Autodesk Inventor part; units mm, degrees
(part 8 of 16)
  spline S46 degree 3 poles (26.1268, 48.1258) (26.0078, 48.1893) (25.8897, 48.2544) (25.7727, 48.3215) (25.7094, 48.3577) (25.6465, 48.3945) (25.5839, 48.4318) (25.5246, 48.4672) (25.4656, 48.5031) (25.407, 48.5395) (25.3517, 48.5739) (25.2966, 48.6087) (25.2419, 48.6441) (25.1905, 48.6773) (25.1393, 48.711) (25.0884, 48.7451) (25.0408, 48.7771) (24.9935, 48.8095) (24.9464, 48.8423) (24.9026, 48.8729) (24.859, 48.9039) (24.8156, 48.9352) (24.7755, 48.9643) (24.7356, 48.9937) (24.6959, 49.0235) (24.6594, 49.051) (24.6231, 49.0788) (24.5871, 49.1069) (24.5541, 49.1326) (24.5213, 49.1586) (24.4888, 49.1849) (24.4593, 49.2088) (24.43, 49.2329) (24.401, 49.2573) (24.3749, 49.2791) (24.349, 49.3012) (24.3233, 49.3236) (24.2894, 49.3531) (24.2559, 49.3832) (24.2226, 49.4135) (24.2152, 49.4202) (24.2077, 49.427) (24.2002, 49.4338) (24.1929, 49.4403) (24.1855, 49.4468) (24.178, 49.4532) (24.1707, 49.4595) (24.1634, 49.4657) (24.156, 49.4719) (24.1487, 49.4779) (24.1414, 49.4839) (24.1341, 49.4898) (24.1268, 49.4956) (24.1195, 49.5013) (24.1122, 49.5069) (24.105, 49.5125) (24.0977, 49.518) (24.0903, 49.5234) (24.0831, 49.5287) (24.0757, 49.5339) (24.0684, 49.5391) (24.061, 49.5442) (24.0537, 49.5492) (24.0462, 49.5541) (24.0388, 49.559) (24.0313, 49.5638) (24.0238, 49.5685) (24.0162, 49.5732) (24.0086, 49.5778) (24.0009, 49.5823) (23.9931, 49.5868) (23.9853, 49.5912) (23.9774, 49.5955) (23.9693, 49.5998) (23.9612, 49.604) (23.953, 49.608) (23.9445, 49.6122) (23.936, 49.6162) (23.9274, 49.6199) (23.9184, 49.6239) (23.9093, 49.6276) (23.9002, 49.6312) (23.8906, 49.6349) (23.8808, 49.6384) (23.871, 49.6416) (23.8605, 49.645) (23.8498, 49.6481) (23.8391, 49.6509) (23.8275, 49.654) (23.8157, 49.6566) (23.8039, 49.6588) (23.7908, 49.6612) (23.7777, 49.6632) (23.7645, 49.6645) (23.7498, 49.666) (23.735, 49.6669) (23.7201, 49.667) (23.7035, 49.6671) (23.6868, 49.6663) (23.6703, 49.6646) (23.6516, 49.6626) (23.6331, 49.6595) (23.6149, 49.6552) (23.5947, 49.6504) (23.5748, 49.6441) (23.5555, 49.6364) (23.5345, 49.628) (23.5141, 49.6181) (23.4949, 49.6064) (23.4765, 49.5952) (23.4591, 49.5824) (23.4419, 49.5693) (23.3571, 49.5047) (23.2781, 49.4332) (23.1957, 49.3657) (23.1134, 49.2982) (23.0277, 49.2348) (22.9477, 49.1643) (22.9315, 49.15) (22.9156, 49.1355) (22.901, 49.1197) (22.8857, 49.1031) (22.872, 49.0851) (22.8597, 49.0661) (22.8483, 49.0487) (22.8383, 49.0304) (22.8296, 49.0115) (22.8217, 48.9945) (22.815, 48.977) (22.8095, 48.9591) (22.8045, 48.9432) (22.8005, 48.927) (22.7973, 48.9107) (22.7945, 48.8961) (22.7924, 48.8815) (22.791, 48.8667) (22.7898, 48.8535) (22.7891, 48.8402) (22.7889, 48.827) (22.7887, 48.8149) (22.789, 48.8029) (22.7897, 48.7909) (22.7903, 48.7798) (22.7913, 48.7688) (22.7926, 48.7578) (22.7938, 48.7475) (22.7953, 48.7373) (22.7971, 48.7271) (22.7987, 48.7175) (22.8006, 48.7078) (22.8027, 48.6983) (22.8048, 48.6891) (22.807, 48.6799) (22.8094, 48.6708) (22.8117, 48.662) (22.8142, 48.6532) (22.8169, 48.6444) (22.8195, 48.6358) (22.8223, 48.6273) (22.8252, 48.6188) (22.8281, 48.6103) (22.8311, 48.602) (22.8342, 48.5936) (22.8373, 48.5853) (22.8406, 48.577) (22.8439, 48.5688) (22.8473, 48.5605) (22.8508, 48.5523) (22.8543, 48.5441) (22.8579, 48.5359) (22.8616, 48.5277) (22.8654, 48.5195) (22.8693, 48.5113) (22.8732, 48.503) (22.8772, 48.4948) (22.8813, 48.4865) (22.8855, 48.4783) (22.8898, 48.47) (22.8941, 48.4616) (22.8985, 48.4533) (22.903, 48.445) (22.9076, 48.4365) (22.9123, 48.4281) (22.917, 48.4197) (22.9218, 48.4112) (22.9267, 48.4026) (22.9317, 48.3941) (22.9368, 48.3855) (22.942, 48.3769) (22.9472, 48.3682) (22.9704, 48.3297) (22.9933, 48.2909) (23.0156, 48.2518) (23.0324, 48.2223) (23.049, 48.1925) (23.0653, 48.1626) (23.0835, 48.1294) (23.1014, 48.0959) (23.119, 48.0623) (23.1384, 48.0253) (23.1575, 47.988) (23.1762, 47.9506) (23.1967, 47.9098) (23.2168, 47.8687) (23.2366, 47.8275) (23.258, 47.7828) (23.279, 47.7379) (23.2997, 47.6928) (23.3219, 47.6442) (23.3437, 47.5953) (23.3651, 47.5463) (23.388, 47.4937) (23.4105, 47.4409) (23.4325, 47.388) (23.456, 47.3314) (23.4789, 47.2746) (23.5014, 47.2176) (23.5253, 47.1571) (23.5487, 47.0962) (23.5715, 47.0352) (23.5957, 46.9706) (23.6193, 46.9057) (23.6423, 46.8407) (23.6667, 46.7719) (23.6904, 46.703) (23.7135, 46.6338) (23.7562, 46.5059) (23.7969, 46.3773) (23.8357, 46.2482) knots 0 0 0 0 0.057795 0.057795 0.057795 0.089038 0.089038 0.089038 0.118617 0.118617 0.118617 0.14653 0.14653 0.14653 0.172778 0.172778 0.172778 0.19736 0.19736 0.19736 0.220277 0.220277 0.220277 0.241529 0.241529 0.241529 0.261115 0.261115 0.261115 0.279036 0.279036 0.279036 0.295292 0.295292 0.295292 0.309882 0.309882 0.309882 0.329164 0.329164 0.329164 0.333477 0.333477 0.333477 0.337694 0.337694 0.337694 0.34182 0.34182 0.34182 0.345864 0.345864 0.345864 0.349834 0.349834 0.349834 0.353742 0.353742 0.353742 0.3576 0.3576 0.3576 0.361424 0.361424 0.361424 0.365232 0.365232 0.365232 0.369048 0.369048 0.369048 0.372899 0.372899 0.372899 0.376819 0.376819 0.376819 0.380853 0.380853 0.380853 0.385052 0.385052 0.385052 0.389482 0.389482 0.389482 0.394225 0.394225 0.394225 0.399381 0.399381 0.399381 0.405067 0.405067 0.405067 0.411413 0.411413 0.411413 0.418548 0.418548 0.418548 0.426565 0.426565 0.426565 0.435472 0.435472 0.435472 0.445133 0.445133 0.445133 0.45436 0.45436 0.45436 0.5 0.5 0.5 0.54564 0.54564 0.54564 0.554867 0.554867 0.554867 0.564528 0.564528 0.564528 0.573435 0.573435 0.573435 0.581452 0.581452 0.581452 0.588587 0.588587 0.588587 0.594933 0.594933 0.594933 0.600619 0.600619 0.600619 0.605775 0.605775 0.605775 0.610518 0.610518 0.610518 0.614948 0.614948 0.614948 0.619147 0.619147 0.619147 0.623181 0.623181 0.623181 0.627101 0.627101 0.627101 0.630952 0.630952 0.630952 0.634768 0.634768 0.634768 0.638576 0.638576 0.638576 0.6424 0.6424 0.6424 0.646258 0.646258 0.646258 0.650166 0.650166 0.650166 0.654136 0.654136 0.654136 0.65818 0.65818 0.65818 0.662306 0.662306 0.662306 0.666523 0.666523 0.666523 0.670836 0.670836 0.670836 0.690118 0.690118 0.690118 0.704708 0.704708 0.704708 0.720964 0.720964 0.720964 0.738885 0.738885 0.738885 0.758471 0.758471 0.758471 0.779723 0.779723 0.779723 0.80264 0.80264 0.80264 0.827222 0.827222 0.827222 0.85347 0.85347 0.85347 0.881383 0.881383 0.881383 0.910962 0.910962 0.910962 0.942205 0.942205 0.942205 1 1 1 1
  arc A248 (26.1268, 48.1258) -> (26.9842, 48.907) centre (0.0435, 77.6158) ccw
  spline S47 degree 3 poles (29.0665, 51.0139) (28.9415, 51.0645) (28.8172, 51.1169) (28.6938, 51.1714) (28.6271, 51.2008) (28.5607, 51.2308) (28.4945, 51.2614) (28.4319, 51.2904) (28.3695, 51.3199) (28.3073, 51.35) (28.2487, 51.3784) (28.1903, 51.4073) (28.1322, 51.4367) (28.0776, 51.4644) (28.0232, 51.4925) (27.969, 51.5212) (27.9183, 51.548) (27.8679, 51.5753) (27.8176, 51.603) (27.7708, 51.6288) (27.7242, 51.6551) (27.6779, 51.6817) (27.6349, 51.7065) (27.5921, 51.7316) (27.5496, 51.7571) (27.5104, 51.7806) (27.4714, 51.8044) (27.4326, 51.8286) (27.3971, 51.8507) (27.3618, 51.8731) (27.3267, 51.8959) (27.2949, 51.9165) (27.2633, 51.9375) (27.2318, 51.9587) (27.2036, 51.9777) (27.1755, 51.9969) (27.1476, 52.0165) (27.1108, 52.0423) (27.0743, 52.0687) (27.0381, 52.0954) (27.03, 52.1013) (27.0219, 52.1073) (27.0137, 52.1132) (27.0057, 52.119) (26.9977, 52.1246) (26.9896, 52.1302) (26.9817, 52.1357) (26.9737, 52.1412) (26.9657, 52.1465) (26.9579, 52.1517) (26.95, 52.1569) (26.9421, 52.162) (26.9343, 52.167) (26.9264, 52.1719) (26.9185, 52.1768) (26.9107, 52.1815) (26.9029, 52.1862) (26.895, 52.1908) (26.8873, 52.1954) (26.8794, 52.1998) (26.8716, 52.2042) (26.8637, 52.2085) (26.8559, 52.2127) (26.848, 52.2168) (26.8401, 52.2209) (26.8321, 52.2249) (26.8241, 52.2288) (26.8161, 52.2327) (26.8081, 52.2365) (26.7999, 52.2401) (26.7917, 52.2438) (26.7835, 52.2473) (26.7752, 52.2507) (26.7667, 52.2542) (26.7582, 52.2575) (26.7496, 52.2607) (26.7407, 52.2639) (26.7318, 52.267) (26.7229, 52.2699) (26.7136, 52.2728) (26.7042, 52.2756) (26.6947, 52.2782) (26.6847, 52.2809) (26.6747, 52.2833) (26.6645, 52.2855) (26.6537, 52.2878) (26.6428, 52.2898) (26.6319, 52.2914) (26.62, 52.2932) (26.608, 52.2946) (26.596, 52.2956) (26.5828, 52.2967) (26.5695, 52.2972) (26.5563, 52.2972) (26.5414, 52.2971) (26.5266, 52.2964) (26.5119, 52.295) (26.4953, 52.2934) (26.4788, 52.2908) (26.4625, 52.2874) (26.4442, 52.2835) (26.4261, 52.2784) (26.4085, 52.2722) (26.3889, 52.2653) (26.3697, 52.257) (26.3513, 52.2473) (26.3313, 52.2368) (26.3121, 52.2248) (26.2942, 52.2111) (26.2771, 52.1981) (26.2611, 52.1836) (26.2454, 52.1688) (26.1678, 52.0957) (26.0967, 52.0163) (26.0218, 51.9406) (25.947, 51.8648) (25.8684, 51.7928) (25.7962, 51.7143) (25.7816, 51.6984) (25.7673, 51.6823) (25.7545, 51.665) (25.741, 51.6469) (25.7292, 51.6276) (25.7189, 51.6075) (25.7095, 51.5889) (25.7014, 51.5697) (25.6947, 51.55) (25.6887, 51.5323) (25.6839, 51.5142) (25.6802, 51.4958) (25.6769, 51.4795) (25.6746, 51.463) (25.6732, 51.4464) (25.6719, 51.4316) (25.6714, 51.4168) (25.6715, 51.402) (25.6716, 51.3887) (25.6723, 51.3754) (25.6735, 51.3622) (25.6746, 51.3502) (25.6762, 51.3383) (25.6781, 51.3264) (25.6799, 51.3155) (25.682, 51.3046) (25.6845, 51.2938) (25.6867, 51.2837) (25.6893, 51.2737) (25.6921, 51.2638) (25.6948, 51.2543) (25.6977, 51.245) (25.7008, 51.2357) (25.7037, 51.2267) (25.7069, 51.2179) (25.7103, 51.2091) (25.7135, 51.2005) (25.7169, 51.192) (25.7205, 51.1836) (25.724, 51.1753) (25.7276, 51.1671) (25.7314, 51.159) (25.7351, 51.1509) (25.739, 51.1429) (25.743, 51.1349) (25.747, 51.1269) (25.7511, 51.1191) (25.7553, 51.1112) (25.7595, 51.1034) (25.7638, 51.0955) (25.7682, 51.0878) (25.7726, 51.08) (25.7772, 51.0722) (25.7818, 51.0645) (25.7865, 51.0566) (25.7913, 51.0489) (25.7961, 51.0411) (25.8011, 51.0333) (25.8061, 51.0255) (25.8112, 51.0178) (25.8164, 51.0099) (25.8216, 51.0021) (25.827, 50.9943) (25.8324, 50.9863) (25.8379, 50.9784) (25.8435, 50.9706) (25.8492, 50.9626) (25.855, 50.9546) (25.8608, 50.9467) (25.8668, 50.9386) (25.8729, 50.9306) (25.8789, 50.9225) (25.906, 50.8866) (25.9328, 50.8505) (25.9591, 50.8139) (25.979, 50.7863) (25.9986, 50.7584) (26.0179, 50.7304) (26.0395, 50.6992) (26.0608, 50.6678) (26.0818, 50.6363) (26.105, 50.6014) (26.1278, 50.5664) (26.1503, 50.5312) (26.175, 50.4927) (26.1993, 50.454) (26.2232, 50.415) (26.2492, 50.3728) (26.2748, 50.3303) (26.3001, 50.2876) (26.3273, 50.2416) (26.3541, 50.1953) (26.3804, 50.1488) (26.4088, 50.0989) (26.4366, 50.0488) (26.464, 49.9984) (26.4933, 49.9446) (26.5221, 49.8905) (26.5504, 49.8362) (26.5805, 49.7784) (26.6101, 49.7204) (26.6392, 49.6621) (26.67, 49.6003) (26.7002, 49.5383) (26.7299, 49.476) (26.7613, 49.4102) (26.7921, 49.3441) (26.8223, 49.2777) (26.8782, 49.155) (26.9321, 49.0314) (26.9842, 48.907) knots 0 0 0 0 0.057795 0.057795 0.057795 0.089038 0.089038 0.089038 0.118617 0.118617 0.118617 0.14653 0.14653 0.14653 0.172778 0.172778 0.172778 0.19736 0.19736 0.19736 0.220277 0.220277 0.220277 0.241529 0.241529 0.241529 0.261115 0.261115 0.261115 0.279036 0.279036 0.279036 0.295292 0.295292 0.295292 0.309882 0.309882 0.309882 0.329164 0.329164 0.329164 0.333477 0.333477 0.333477 0.337694 0.337694 0.337694 0.34182 0.34182 0.34182 0.345864 0.345864 0.345864 0.349834 0.349834 0.349834 0.353742 0.353742 0.353742 0.3576 0.3576 0.3576 0.361424 0.361424 0.361424 0.365232 0.365232 0.365232 0.369048 0.369048 0.369048 0.372899 0.372899 0.372899 0.376819 0.376819 0.376819 0.380853 0.380853 0.380853 0.385052 0.385052 0.385052 0.389482 0.389482 0.389482 0.394225 0.394225 0.394225 0.399381 0.399381 0.399381 0.405067 0.405067 0.405067 0.411413 0.411413 0.411413 0.418548 0.418548 0.418548 0.426565 0.426565 0.426565 0.435472 0.435472 0.435472 0.445133 0.445133 0.445133 0.45436 0.45436 0.45436 0.5 0.5 0.5 0.54564 0.54564 0.54564 0.554867 0.554867 0.554867 0.564528 0.564528 0.564528 0.573435 0.573435 0.573435 0.581452 0.581452 0.581452 0.588587 0.588587 0.588587 0.594933 0.594933 0.594933 0.600619 0.600619 0.600619 0.605775 0.605775 0.605775 0.610518 0.610518 0.610518 0.614948 0.614948 0.614948 0.619147 0.619147 0.619147 0.623181 0.623181 0.623181 0.627101 0.627101 0.627101 0.630952 0.630952 0.630952 0.634768 0.634768 0.634768 0.638576 0.638576 0.638576 0.6424 0.6424 0.6424 0.646258 0.646258 0.646258 0.650166 0.650166 0.650166 0.654136 0.654136 0.654136 0.65818 0.65818 0.65818 0.662306 0.662306 0.662306 0.666523 0.666523 0.666523 0.670836 0.670836 0.670836 0.690118 0.690118 0.690118 0.704708 0.704708 0.704708 0.720964 0.720964 0.720964 0.738885 0.738885 0.738885 0.758471 0.758471 0.758471 0.779723 0.779723 0.779723 0.80264 0.80264 0.80264 0.827222 0.827222 0.827222 0.85347 0.85347 0.85347 0.881383 0.881383 0.881383 0.910962 0.910962 0.910962 0.942205 0.942205 0.942205 1 1 1 1
  arc A249 (29.0665, 51.0139) -> (29.8375, 51.8803) centre (0.0435, 77.6158) ccw
  spline S48 degree 3 poles (31.6882, 54.1933) (31.5586, 54.2306) (31.4295, 54.2698) (31.3011, 54.311) (31.2317, 54.3333) (31.1624, 54.3562) (31.0934, 54.3797) (31.0281, 54.402) (30.963, 54.4248) (30.898, 54.4483) (30.8368, 54.4704) (30.7757, 54.493) (30.7148, 54.5162) (30.6576, 54.538) (30.6005, 54.5603) (30.5437, 54.5831) (30.4905, 54.6045) (30.4374, 54.6263) (30.3846, 54.6487) (30.3353, 54.6695) (30.2862, 54.6907) (30.2373, 54.7124) (30.192, 54.7325) (30.1468, 54.753) (30.1019, 54.7739) (30.0604, 54.7932) (30.0191, 54.8128) (29.9781, 54.8328) (29.9404, 54.8511) (29.903, 54.8697) (29.8657, 54.8887) (29.8319, 54.9059) (29.7983, 54.9234) (29.7648, 54.9412) (29.7347, 54.9571) (29.7048, 54.9734) (29.675, 54.9899) (29.6357, 55.0117) (29.5966, 55.0342) (29.5578, 55.0569) (29.5491, 55.062) (29.5404, 55.0671) (29.5317, 55.0721) (29.5232, 55.077) (29.5146, 55.0818) (29.506, 55.0865) (29.4975, 55.0911) (29.489, 55.0957) (29.4805, 55.1002) (29.4722, 55.1046) (29.4638, 55.1089) (29.4553, 55.1131) (29.4471, 55.1173) (29.4387, 55.1214) (29.4304, 55.1253) (29.4222, 55.1293) (29.4139, 55.1331) (29.4056, 55.1369) (29.3974, 55.1406) (29.3891, 55.1442) (29.3808, 55.1477) (29.3726, 55.1512) (29.3643, 55.1545) (29.356, 55.1578) (29.3478, 55.1611) (29.3395, 55.1642) (29.3311, 55.1672) (29.3227, 55.1702) (29.3143, 55.1732) (29.3059, 55.1759) (29.2973, 55.1787) (29.2887, 55.1814) (29.2801, 55.1839) (29.2713, 55.1865) (29.2625, 55.1889) (29.2536, 55.1911) (29.2445, 55.1934) (29.2353, 55.1955) (29.2261, 55.1975) (29.2165, 55.1995) (29.2069, 55.2012) (29.1972, 55.2028) (29.187, 55.2044) (29.1767, 55.2058) (29.1665, 55.2069) (29.1554, 55.2081) (29.1444, 55.2089) (29.1333, 55.2094) (29.1213, 55.21) (29.1093, 55.2101) (29.0973, 55.2098) (29.084, 55.2095) (29.0707, 55.2086) (29.0575, 55.2072) (29.0428, 55.2056) (29.0281, 55.2034) (29.0136, 55.2004) (28.9973, 55.197) (28.9812, 55.1928) (28.9653, 55.1877) (28.9475, 55.1819) (28.9301, 55.175) (28.9132, 55.167) (28.8944, 55.158) (28.8762, 55.1478) (28.8589, 55.1362) (28.8401, 55.1237) (28.8223, 55.1097) (28.8059, 55.0942) (28.7902, 55.0795) (28.7759, 55.0634) (28.7618, 55.047) (28.6923, 54.9662) (28.6298, 54.8798) (28.5633, 54.7967) (28.4968, 54.7135) (28.4262, 54.6337) (28.3626, 54.5481) (28.3497, 54.5308) (28.3372, 54.5132) (28.3262, 54.4947) (28.3147, 54.4753) (28.305, 54.4549) (28.2969, 54.4338) (28.2894, 54.4143) (28.2834, 54.3944) (28.2788, 54.3741) (28.2747, 54.3558) (28.2718, 54.3373) (28.27, 54.3187) (28.2685, 54.3021) (28.2679, 54.2854) (28.2682, 54.2687) (28.2685, 54.2539) (28.2695, 54.2391) (28.2712, 54.2244) (28.2727, 54.2112) (28.2748, 54.1981) (28.2774, 54.1851) (28.2797, 54.1733) (28.2825, 54.1616) (28.2857, 54.15) (28.2886, 54.1393) (28.2918, 54.1287) (28.2954, 54.1182) (28.2987, 54.1084) (28.3023, 54.0987) (28.3061, 54.0891) (28.3098, 54.08) (28.3136, 54.071) (28.3177, 54.0621) (28.3216, 54.0535) (28.3257, 54.045) (28.3299, 54.0366) (28.334, 54.0285) (28.3383, 54.0204) (28.3427, 54.0124) (28.3471, 54.0045) (28.3516, 53.9967) (28.3562, 53.989) (28.3607, 53.9814) (28.3654, 53.9738) (28.3702, 53.9663) (28.375, 53.9588) (28.3799, 53.9514) (28.3849, 53.944) (28.3899, 53.9366) (28.395, 53.9293) (28.4002, 53.9221) (28.4054, 53.9147) (28.4108, 53.9075) (28.4162, 53.9003) (28.4217, 53.893) (28.4272, 53.8858) (28.4329, 53.8786) (28.4386, 53.8713) (28.4444, 53.8641) (28.4503, 53.8569) (28.4562, 53.8496) (28.4623, 53.8424) (28.4684, 53.8352) (28.4747, 53.8279) (28.481, 53.8206) (28.4873, 53.8134) (28.4939, 53.806) (28.5004, 53.7987) (28.5071, 53.7914) (28.5139, 53.784) (28.5207, 53.7767) (28.5276, 53.7693) (28.5583, 53.7364) (28.5887, 53.7033) (28.6187, 53.6697) (28.6413, 53.6443) (28.6637, 53.6186) (28.6859, 53.5928) (28.7106, 53.564) (28.7351, 53.535) (28.7593, 53.5058) (28.786, 53.4736) (28.8123, 53.4411) (28.8384, 53.4085) (28.867, 53.3728) (28.8952, 53.3368) (28.9231, 53.3006) (28.9533, 53.2613) (28.9832, 53.2217) (29.0128, 53.1819) (29.0447, 53.139) (29.0761, 53.0957) (29.1072, 53.0522) (29.1406, 53.0056) (29.1736, 52.9586) (29.2061, 52.9114) (29.2408, 52.8609) (29.2751, 52.8102) (29.3089, 52.7591) (29.3449, 52.7048) (29.3804, 52.6502) (29.4154, 52.5952) (29.4525, 52.537) (29.4891, 52.4785) (29.5251, 52.4196) (29.5632, 52.3575) (29.6008, 52.295) (29.6377, 52.2321) (29.7061, 52.1159) (29.7727, 51.9986) (29.8375, 51.8803) knots 0 0 0 0 0.057795 0.057795 0.057795 0.089038 0.089038 0.089038 0.118617 0.118617 0.118617 0.14653 0.14653 0.14653 0.172778 0.172778 0.172778 0.19736 0.19736 0.19736 0.220277 0.220277 0.220277 0.241529 0.241529 0.241529 0.261115 0.261115 0.261115 0.279036 0.279036 0.279036 0.295292 0.295292 0.295292 0.309882 0.309882 0.309882 0.329164 0.329164 0.329164 0.333477 0.333477 0.333477 0.337694 0.337694 0.337694 0.34182 0.34182 0.34182 0.345864 0.345864 0.345864 0.349834 0.349834 0.349834 0.353742 0.353742 0.353742 0.3576 0.3576 0.3576 0.361424 0.361424 0.361424 0.365232 0.365232 0.365232 0.369048 0.369048 0.369048 0.372899 0.372899 0.372899 0.376819 0.376819 0.376819 0.380853 0.380853 0.380853 0.385052 0.385052 0.385052 0.389482 0.389482 0.389482 0.394225 0.394225 0.394225 0.399381 0.399381 0.399381 0.405067 0.405067 0.405067 0.411413 0.411413 0.411413 0.418548 0.418548 0.418548 0.426565 0.426565 0.426565 0.435472 0.435472 0.435472 0.445133 0.445133 0.445133 0.45436 0.45436 0.45436 0.5 0.5 0.5 0.54564 0.54564 0.54564 0.554867 0.554867 0.554867 0.564528 0.564528 0.564528 0.573435 0.573435 0.573435 0.581452 0.581452 0.581452 0.588587 0.588587 0.588587 0.594933 0.594933 0.594933 0.600619 0.600619 0.600619 0.605775 0.605775 0.605775 0.610518 0.610518 0.610518 0.614948 0.614948 0.614948 0.619147 0.619147 0.619147 0.623181 0.623181 0.623181 0.627101 0.627101 0.627101 0.630952 0.630952 0.630952 0.634768 0.634768 0.634768 0.638576 0.638576 0.638576 0.6424 0.6424 0.6424 0.646258 0.646258 0.646258 0.650166 0.650166 0.650166 0.654136 0.654136 0.654136 0.65818 0.65818 0.65818 0.662306 0.662306 0.662306 0.666523 0.666523 0.666523 0.670836 0.670836 0.670836 0.690118 0.690118 0.690118 0.704708 0.704708 0.704708 0.720964 0.720964 0.720964 0.738885 0.738885 0.738885 0.758471 0.758471 0.758471 0.779723 0.779723 0.779723 0.80264 0.80264 0.80264 0.827222 0.827222 0.827222 0.85347 0.85347 0.85347 0.881383 0.881383 0.881383 0.910962 0.910962 0.910962 0.942205 0.942205 0.942205 1 1 1 1
  arc A250 (31.6882, 54.1933) -> (32.3644, 55.1356) centre (0.0435, 77.6158) ccw
  spline S49 degree 3 poles (33.9631, 57.6294) (33.8303, 57.6529) (33.6979, 57.6784) (33.5659, 57.706) (33.4945, 57.7209) (33.4233, 57.7364) (33.3522, 57.7526) (33.2849, 57.7679) (33.2177, 57.7838) (33.1507, 57.8003) (33.0874, 57.8159) (33.0243, 57.8321) (32.9614, 57.8488) (32.9022, 57.8645) (32.8431, 57.8807) (32.7842, 57.8975) (32.729, 57.9131) (32.674, 57.9293) (32.6191, 57.946) (32.5679, 57.9615) (32.5169, 57.9775) (32.466, 57.994) (32.4188, 58.0092) (32.3717, 58.0249) (32.3248, 58.041) (32.2816, 58.0558) (32.2385, 58.071) (32.1955, 58.0866) (32.1562, 58.1009) (32.117, 58.1155) (32.078, 58.1304) (32.0426, 58.144) (32.0073, 58.1579) (31.9721, 58.1721) (31.9405, 58.1848) (31.909, 58.1978) (31.8777, 58.2112) (31.8363, 58.2288) (31.7952, 58.247) (31.7542, 58.2655) (31.745, 58.2697) (31.7358, 58.2739) (31.7266, 58.2779) (31.7176, 58.2819) (31.7086, 58.2858) (31.6995, 58.2896) (31.6906, 58.2933) (31.6817, 58.297) (31.6728, 58.3005) (31.664, 58.304) (31.6552, 58.3074) (31.6464, 58.3108) (31.6377, 58.314) (31.629, 58.3172) (31.6203, 58.3203) (31.6117, 58.3234) (31.6031, 58.3263) (31.5944, 58.3292) (31.5859, 58.332) (31.5773, 58.3347) (31.5687, 58.3373) (31.5601, 58.3399) (31.5516, 58.3424) (31.543, 58.3448) (31.5344, 58.3472) (31.5258, 58.3494) (31.5172, 58.3516) (31.5085, 58.3537) (31.4999, 58.3557) (31.4912, 58.3576) (31.4824, 58.3595) (31.4736, 58.3613) (31.4647, 58.3629) (31.4557, 58.3645) (31.4467, 58.366) (31.4376, 58.3673) (31.4283, 58.3686) (31.419, 58.3697) (31.4096, 58.3707) (31.3998, 58.3717) (31.3901, 58.3724) (31.3803, 58.373) (31.37, 58.3735) (31.3596, 58.3738) (31.3493, 58.3738) (31.3382, 58.3738) (31.3271, 58.3735) (31.3161, 58.3729) (31.3041, 58.3722) (31.2921, 58.371) (31.2802, 58.3695) (31.267, 58.3678) (31.2539, 58.3655) (31.2409, 58.3627) (31.2264, 58.3596) (31.2121, 58.3559) (31.198, 58.3514) (31.1821, 58.3464) (31.1665, 58.3405) (31.1513, 58.3337) (31.1342, 58.3261) (31.1175, 58.3174) (31.1016, 58.3076) (31.0838, 58.2968) (31.0668, 58.2847) (31.0508, 58.2714) (31.0334, 58.257) (31.0172, 58.2412) (31.0025, 58.2241) (30.9884, 58.2078) (30.9758, 58.1903) (30.9636, 58.1725) (30.9029, 58.0849) (30.8498, 57.9924) (30.7923, 57.9028) (30.7348, 57.8132) (30.673, 57.7264) (30.6187, 57.6346) (30.6077, 57.616) (30.597, 57.5973) (30.5881, 57.5777) (30.5787, 57.5572) (30.5711, 57.5359) (30.5653, 57.514) (30.5599, 57.4939) (30.556, 57.4735) (30.5535, 57.4528) (30.5513, 57.4342) (30.5504, 57.4155) (30.5506, 57.3968) (30.5508, 57.3801) (30.552, 57.3635) (30.554, 57.3469) (30.5559, 57.3322) (30.5584, 57.3176) (30.5616, 57.3032) (30.5645, 57.2902) (30.5679, 57.2774) (30.5719, 57.2647) (30.5754, 57.2532) (30.5794, 57.2418) (30.5838, 57.2306) (30.5878, 57.2203) (30.5922, 57.2101) (30.5968, 57.2001) (30.6011, 57.1907) (30.6057, 57.1814) (30.6105, 57.1723) (30.6151, 57.1636) (30.6199, 57.155) (30.6248, 57.1466) (30.6296, 57.1385) (30.6345, 57.1305) (30.6396, 57.1225) (30.6446, 57.1149) (30.6497, 57.1073) (30.6549, 57.0998) (30.6601, 57.0924) (30.6654, 57.0851) (30.6707, 57.0779) (30.6761, 57.0708) (30.6815, 57.0638) (30.6871, 57.0568) (30.6926, 57.0498) (30.6983, 57.043) (30.704, 57.0362) (30.7098, 57.0294) (30.7156, 57.0226) (30.7215, 57.0159) (30.7275, 57.0092) (30.7336, 57.0026) (30.7397, 56.996) (30.7459, 56.9893) (30.7522, 56.9827) (30.7585, 56.9761) (30.765, 56.9695) (30.7715, 56.9629) (30.7781, 56.9564) (30.7848, 56.9498) (30.7916, 56.9432) (30.7984, 56.9367) (30.8054, 56.9301) (30.8125, 56.9235) (30.8196, 56.917) (30.8268, 56.9103) (30.8341, 56.9037) (30.8415, 56.8972) (30.849, 56.8905) (30.8566, 56.8839) (30.8642, 56.8773) (30.8982, 56.8478) (30.9319, 56.818) (30.9652, 56.7878) (30.9904, 56.7649) (31.0153, 56.7417) (31.0401, 56.7183) (31.0677, 56.6923) (31.095, 56.666) (31.1221, 56.6395) (31.152, 56.6102) (31.1817, 56.5807) (31.2111, 56.551) (31.2432, 56.5184) (31.275, 56.4856) (31.3065, 56.4525) (31.3407, 56.4166) (31.3746, 56.3804) (31.4081, 56.3439) (31.4443, 56.3045) (31.4801, 56.2648) (31.5156, 56.2248) (31.5537, 56.1819) (31.5914, 56.1386) (31.6286, 56.095) (31.6685, 56.0485) (31.7079, 56.0016) (31.7469, 55.9543) (31.7883, 55.9041) (31.8293, 55.8535) (31.8699, 55.8025) (31.9129, 55.7485) (31.9553, 55.6941) (31.9974, 55.6393) (32.0417, 55.5815) (32.0856, 55.5233) (32.1289, 55.4646) (32.2091, 55.3562) (32.2875, 55.2465) (32.3644, 55.1356) knots 0 0 0 0 0.057795 0.057795 0.057795 0.089038 0.089038 0.089038 0.118617 0.118617 0.118617 0.14653 0.14653 0.14653 0.172778 0.172778 0.172778 0.19736 0.19736 0.19736 0.220277 0.220277 0.220277 0.241529 0.241529 0.241529 0.261115 0.261115 0.261115 0.279036 0.279036 0.279036 0.295292 0.295292 0.295292 0.309882 0.309882 0.309882 0.329164 0.329164 0.329164 0.333477 0.333477 0.333477 0.337694 0.337694 0.337694 0.34182 0.34182 0.34182 0.345864 0.345864 0.345864 0.349834 0.349834 0.349834 0.353742 0.353742 0.353742 0.3576 0.3576 0.3576 0.361424 0.361424 0.361424 0.365232 0.365232 0.365232 0.369048 0.369048 0.369048 0.372899 0.372899 0.372899 0.376819 0.376819 0.376819 0.380853 0.380853 0.380853 0.385052 0.385052 0.385052 0.389482 0.389482 0.389482 0.394225 0.394225 0.394225 0.399381 0.399381 0.399381 0.405067 0.405067 0.405067 0.411413 0.411413 0.411413 0.418548 0.418548 0.418548 0.426565 0.426565 0.426565 0.435472 0.435472 0.435472 0.445133 0.445133 0.445133 0.45436 0.45436 0.45436 0.5 0.5 0.5 0.54564 0.54564 0.54564 0.554867 0.554867 0.554867 0.564528 0.564528 0.564528 0.573435 0.573435 0.573435 0.581452 0.581452 0.581452 0.588587 0.588587 0.588587 0.594933 0.594933 0.594933 0.600619 0.600619 0.600619 0.605775 0.605775 0.605775 0.610518 0.610518 0.610518 0.614948 0.614948 0.614948 0.619147 0.619147 0.619147 0.623181 0.623181 0.623181 0.627101 0.627101 0.627101 0.630952 0.630952 0.630952 0.634768 0.634768 0.634768 0.638576 0.638576 0.638576 0.6424 0.6424 0.6424 0.646258 0.646258 0.646258 0.650166 0.650166 0.650166 0.654136 0.654136 0.654136 0.65818 0.65818 0.65818 0.662306 0.662306 0.662306 0.666523 0.666523 0.666523 0.670836 0.670836 0.670836 0.690118 0.690118 0.690118 0.704708 0.704708 0.704708 0.720964 0.720964 0.720964 0.738885 0.738885 0.738885 0.758471 0.758471 0.758471 0.779723 0.779723 0.779723 0.80264 0.80264 0.80264 0.827222 0.827222 0.827222 0.85347 0.85347 0.85347 0.881383 0.881383 0.881383 0.910962 0.910962 0.910962 0.942205 0.942205 0.942205 1 1 1 1
  arc A251 (33.9631, 57.6294) -> (34.5371, 58.6372) centre (0.0435, 77.6158) ccw
  spline S50 degree 3 poles (35.8665, 61.2844) (35.7319, 61.294) (35.5975, 61.3055) (35.4634, 61.3191) (35.3908, 61.3265) (35.3184, 61.3345) (35.246, 61.3431) (35.1774, 61.3513) (35.109, 61.3601) (35.0406, 61.3695) (34.9761, 61.3784) (34.9116, 61.3879) (34.8473, 61.3979) (34.7867, 61.4073) (34.7263, 61.4173) (34.666, 61.4278) (34.6094, 61.4376) (34.553, 61.448) (34.4967, 61.4588) (34.4442, 61.4689) (34.3917, 61.4795) (34.3394, 61.4905) (34.2909, 61.5008) (34.2425, 61.5114) (34.1941, 61.5225) (34.1496, 61.5328) (34.1051, 61.5434) (34.0608, 61.5544) (34.0202, 61.5645) (33.9797, 61.5749) (33.9393, 61.5857) (33.9026, 61.5955) (33.8661, 61.6056) (33.8296, 61.6161) (33.7969, 61.6254) (33.7642, 61.6351) (33.7317, 61.6451) (33.6886, 61.6583) (33.6458, 61.6721) (33.6031, 61.6862) (33.5936, 61.6894) (33.584, 61.6926) (33.5744, 61.6956) (33.5651, 61.6987) (33.5557, 61.7016) (33.5462, 61.7044) (33.537, 61.7072) (33.5278, 61.7099) (33.5185, 61.7125) (33.5094, 61.7151) (33.5003, 61.7175) (33.4912, 61.7199) (33.4822, 61.7223) (33.4732, 61.7245) (33.4642, 61.7267) (33.4554, 61.7288) (33.4465, 61.7309) (33.4376, 61.7328) (33.4288, 61.7347) (33.42, 61.7365) (33.4111, 61.7382) (33.4024, 61.7399) (33.3936, 61.7415) (33.3848, 61.743) (33.376, 61.7444) (33.3672, 61.7458) (33.3584, 61.747) (33.3496, 61.7482) (33.3408, 61.7493) (33.3319, 61.7503) (33.323, 61.7513) (33.314, 61.7521) (33.3051, 61.7527) (33.2959, 61.7534) (33.2868, 61.7539) (33.2777, 61.7543) (33.2682, 61.7546) (33.2588, 61.7548) (33.2494, 61.7548) (33.2396, 61.7547) (33.2298, 61.7545) (33.22, 61.754) (33.2097, 61.7534) (33.1994, 61.7527) (33.1891, 61.7516) (33.1781, 61.7504) (33.1671, 61.749) (33.1562, 61.7472) (33.1443, 61.7452) (33.1325, 61.7428) (33.1208, 61.74) (33.1079, 61.737) (33.0951, 61.7334) (33.0825, 61.7292) (33.0684, 61.7246) (33.0546, 61.7194) (33.041, 61.7134) (33.0257, 61.7068) (33.0108, 61.6993) (32.9964, 61.691) (32.9802, 61.6816) (32.9645, 61.6712) (32.9497, 61.6599) (32.9331, 61.6472) (32.9175, 61.6334) (32.903, 61.6185) (32.8872, 61.6024) (32.8727, 61.585) (32.8598, 61.5664) (32.8476, 61.5487) (32.8369, 61.53) (32.8266, 61.5111) (32.7753, 61.4176) (32.7322, 61.3201) (32.6844, 61.2249) (32.6366, 61.1298) (32.5842, 61.037) (32.5398, 60.94) (32.5308, 60.9204) (32.5222, 60.9007) (32.5153, 60.8803) (32.5081, 60.8589) (32.5028, 60.8369) (32.4993, 60.8146) (32.496, 60.794) (32.4942, 60.7732) (32.494, 60.7524) (32.4938, 60.7337) (32.4948, 60.715) (32.497, 60.6964) (32.4989, 60.6798) (32.5018, 60.6634) (32.5056, 60.6472) (32.5089, 60.6328) (32.513, 60.6185) (32.5177, 60.6045) (32.5219, 60.5919) (32.5267, 60.5795) (32.5319, 60.5673) (32.5367, 60.5562) (32.5418, 60.5453) (32.5473, 60.5346) (32.5524, 60.5248) (32.5578, 60.5151) (32.5634, 60.5056) (32.5687, 60.4967) (32.5742, 60.488) (32.58, 60.4794) (32.5854, 60.4712) (32.5911, 60.4632) (32.5969, 60.4553) (32.6025, 60.4478) (32.6083, 60.4403) (32.6142, 60.433) (32.6199, 60.4259) (32.6258, 60.4188) (32.6318, 60.4119) (32.6376, 60.4051) (32.6436, 60.3984) (32.6498, 60.3919) (32.6558, 60.3853) (32.662, 60.3789) (32.6682, 60.3725) (32.6745, 60.3662) (32.6808, 60.36) (32.6872, 60.3538) (32.6936, 60.3476) (32.7001, 60.3415) (32.7067, 60.3355) (32.7134, 60.3294) (32.7201, 60.3235) (32.7269, 60.3175) (32.7338, 60.3116) (32.7407, 60.3056) (32.7477, 60.2998) (32.7548, 60.2939) (32.762, 60.288) (32.7692, 60.2822) (32.7766, 60.2763) (32.784, 60.2705) (32.7915, 60.2648) (32.7991, 60.2589) (32.8068, 60.2531) (32.8146, 60.2473) (32.8225, 60.2415) (32.8304, 60.2357) (32.8384, 60.23) (32.8466, 60.2241) (32.8549, 60.2184) (32.8631, 60.2126) (32.9, 60.1868) (32.9366, 60.1607) (32.9729, 60.1341) (33.0004, 60.1139) (33.0276, 60.0935) (33.0547, 60.0728) (33.0848, 60.0498) (33.1148, 60.0265) (33.1445, 60.003) (33.1773, 59.977) (33.2099, 59.9508) (33.2422, 59.9243) (33.2775, 59.8953) (33.3126, 59.8659) (33.3474, 59.8363) (33.3852, 59.8042) (33.4226, 59.7717) (33.4598, 59.7389) (33.4999, 59.7035) (33.5397, 59.6678) (33.5792, 59.6317) (33.6215, 59.593) (33.6635, 59.5539) (33.7052, 59.5145) (33.7496, 59.4723) (33.7937, 59.4298) (33.8374, 59.3869) (33.8839, 59.3413) (33.93, 59.2952) (33.9756, 59.2488) (34.024, 59.1996) (34.072, 59.1499) (34.1195, 59.0998) (34.1697, 59.0469) (34.2194, 58.9936) (34.2686, 58.9398) (34.3597, 58.8403) (34.4491, 58.7394) (34.5371, 58.6372) knots 0 0 0 0 0.057795 0.057795 0.057795 0.089038 0.089038 0.089038 0.118617 0.118617 0.118617 0.14653 0.14653 0.14653 0.172778 0.172778 0.172778 0.19736 0.19736 0.19736 0.220277 0.220277 0.220277 0.241529 0.241529 0.241529 0.261115 0.261115 0.261115 0.279036 0.279036 0.279036 0.295292 0.295292 0.295292 0.309882 0.309882 0.309882 0.329164 0.329164 0.329164 0.333477 0.333477 0.333477 0.337694 0.337694 0.337694 0.34182 0.34182 0.34182 0.345864 0.345864 0.345864 0.349834 0.349834 0.349834 0.353742 0.353742 0.353742 0.3576 0.3576 0.3576 0.361424 0.361424 0.361424 0.365232 0.365232 0.365232 0.369048 0.369048 0.369048 0.372899 0.372899 0.372899 0.376819 0.376819 0.376819 0.380853 0.380853 0.380853 0.385052 0.385052 0.385052 0.389482 0.389482 0.389482 0.394225 0.394225 0.394225 0.399381 0.399381 0.399381 0.405067 0.405067 0.405067 0.411413 0.411413 0.411413 0.418548 0.418548 0.418548 0.426565 0.426565 0.426565 0.435472 0.435472 0.435472 0.445133 0.445133 0.445133 0.45436 0.45436 0.45436 0.5 0.5 0.5 0.54564 0.54564 0.54564 0.554867 0.554867 0.554867 0.564528 0.564528 0.564528 0.573435 0.573435 0.573435 0.581452 0.581452 0.581452 0.588587 0.588587 0.588587 0.594933 0.594933 0.594933 0.600619 0.600619 0.600619 0.605775 0.605775 0.605775 0.610518 0.610518 0.610518 0.614948 0.614948 0.614948 0.619147 0.619147 0.619147 0.623181 0.623181 0.623181 0.627101 0.627101 0.627101 0.630952 0.630952 0.630952 0.634768 0.634768 0.634768 0.638576 0.638576 0.638576 0.6424 0.6424 0.6424 0.646258 0.646258 0.646258 0.650166 0.650166 0.650166 0.654136 0.654136 0.654136 0.65818 0.65818 0.65818 0.662306 0.662306 0.662306 0.666523 0.666523 0.666523 0.670836 0.670836 0.670836 0.690118 0.690118 0.690118 0.704708 0.704708 0.704708 0.720964 0.720964 0.720964 0.738885 0.738885 0.738885 0.758471 0.758471 0.758471 0.779723 0.779723 0.779723 0.80264 0.80264 0.80264 0.827222 0.827222 0.827222 0.85347 0.85347 0.85347 0.881383 0.881383 0.881383 0.910962 0.910962 0.910962 0.942205 0.942205 0.942205 1 1 1 1
  arc A252 (35.8665, 61.2844) -> (36.332, 62.3467) centre (0.0435, 77.6158) ccw
  spline S51 degree 3 poles (37.3773, 65.1184) (37.2425, 65.1138) (37.1077, 65.1112) (36.9728, 65.1108) (36.8999, 65.1105) (36.827, 65.1109) (36.7541, 65.1119) (36.6851, 65.1129) (36.616, 65.1145) (36.5471, 65.1167) (36.482, 65.1188) (36.4169, 65.1215) (36.3518, 65.1247) (36.2906, 65.1278) (36.2295, 65.1314) (36.1684, 65.1355) (36.1112, 65.1394) (36.054, 65.1438) (35.9968, 65.1487) (35.9435, 65.1532) (35.8903, 65.1583) (35.8371, 65.1638) (35.7878, 65.1689) (35.7385, 65.1744) (35.6892, 65.1804) (35.6439, 65.1859) (35.5985, 65.1918) (35.5533, 65.1981) (35.5119, 65.2039) (35.4705, 65.2101) (35.4292, 65.2166) (35.3917, 65.2225) (35.3543, 65.2287) (35.3169, 65.2353) (35.2834, 65.2412) (35.2499, 65.2474) (35.2165, 65.2539) (35.1724, 65.2625) (35.1283, 65.2718) (35.0844, 65.2814) (35.0745, 65.2836) (35.0647, 65.2857) (35.0548, 65.2878) (35.0452, 65.2898) (35.0356, 65.2917) (35.0259, 65.2936) (35.0164, 65.2954) (35.007, 65.2971) (34.9975, 65.2987) (34.9882, 65.3003) (34.9789, 65.3018) (34.9695, 65.3032) (34.9604, 65.3046) (34.9512, 65.3059) (34.942, 65.3072) (34.933, 65.3083) (34.9239, 65.3094) (34.9149, 65.3104) (34.9059, 65.3114) (34.8969, 65.3123) (34.888, 65.3131) (34.8791, 65.3138) (34.8702, 65.3145) (34.8613, 65.315) (34.8524, 65.3156) (34.8435, 65.316) (34.8346, 65.3163) (34.8257, 65.3166) (34.8168, 65.3168) (34.8079, 65.3168) (34.799, 65.3168) (34.79, 65.3167) (34.781, 65.3164) (34.7718, 65.3161) (34.7627, 65.3157) (34.7536, 65.3151) (34.7442, 65.3145) (34.7348, 65.3136) (34.7254, 65.3126) (34.7157, 65.3115) (34.706, 65.3103) (34.6963, 65.3088) (34.6861, 65.3072) (34.6759, 65.3053) (34.6658, 65.3032) (34.655, 65.3009) (34.6442, 65.2983) (34.6335, 65.2953) (34.6219, 65.2921) (34.6104, 65.2885) (34.5991, 65.2845) (34.5866, 65.2801) (34.5742, 65.2752) (34.5621, 65.2698) (34.5486, 65.2637) (34.5354, 65.2571) (34.5225, 65.2497) (34.508, 65.2415) (34.4939, 65.2325) (34.4805, 65.2227) (34.4653, 65.2117) (34.4509, 65.1998) (34.4372, 65.1869) (34.4221, 65.1726) (34.4081, 65.1572) (34.3952, 65.1409) (34.3812, 65.1232) (34.3685, 65.1044) (34.3577, 65.0846) (34.3474, 65.0657) (34.3387, 65.046) (34.3304, 65.0261) (34.2892, 64.9277) (34.2565, 64.8263) (34.2189, 64.7266) (34.1814, 64.627) (34.1389, 64.5292) (34.1049, 64.4282) (34.098, 64.4077) (34.0915, 64.3872) (34.0867, 64.3662) (34.0818, 64.3442) (34.0789, 64.3217) (34.0777, 64.2992) (34.0766, 64.2784) (34.077, 64.2575) (34.0789, 64.2368) (34.0807, 64.2182) (34.0836, 64.1996) (34.0877, 64.1814) (34.0914, 64.1651) (34.096, 64.1491) (34.1014, 64.1334) (34.1063, 64.1194) (34.1118, 64.1056) (34.118, 64.0921) (34.1235, 64.08) (34.1295, 64.0682) (34.136, 64.0566) (34.1419, 64.0461) (34.1481, 64.0358) (34.1547, 64.0258) (34.1608, 64.0165) (34.1672, 64.0075) (34.1738, 63.9986) (34.18, 63.9903) (34.1864, 63.9822) (34.193, 63.9742) (34.1993, 63.9667) (34.2057, 63.9593) (34.2123, 63.9521) (34.2187, 63.9452) (34.2252, 63.9383) (34.2318, 63.9317) (34.2383, 63.9252) (34.2448, 63.9188) (34.2515, 63.9126) (34.2581, 63.9064) (34.2648, 63.9004) (34.2715, 63.8945) (34.2782, 63.8886) (34.285, 63.8829) (34.2919, 63.8772) (34.2988, 63.8716) (34.3057, 63.866) (34.3127, 63.8606) (34.3198, 63.8551) (34.3269, 63.8497) (34.3341, 63.8444) (34.3413, 63.8391) (34.3486, 63.8338) (34.356, 63.8287) (34.3635, 63.8234) (34.371, 63.8183) (34.3786, 63.8132) (34.3863, 63.808) (34.394, 63.803) (34.4018, 63.798) (34.4098, 63.7929) (34.4178, 63.7878) (34.4258, 63.7829) (34.434, 63.7779) (34.4423, 63.7729) (34.4505, 63.768) (34.459, 63.763) (34.4675, 63.7581) (34.4761, 63.7532) (34.4848, 63.7483) (34.4937, 63.7434) (34.5025, 63.7385) (34.5418, 63.7167) (34.581, 63.6946) (34.6199, 63.6719) (34.6493, 63.6547) (34.6785, 63.6373) (34.7076, 63.6195) (34.74, 63.5998) (34.7722, 63.5798) (34.8042, 63.5595) (34.8395, 63.5371) (34.8747, 63.5144) (34.9096, 63.4914) (34.9478, 63.4662) (34.9857, 63.4407) (35.0234, 63.4149) (35.0643, 63.3869) (35.105, 63.3585) (35.1454, 63.3298) (35.189, 63.2988) (35.2323, 63.2674) (35.2753, 63.2357) (35.3215, 63.2016) (35.3673, 63.1671) (35.4129, 63.1322) (35.4615, 63.095) (35.5098, 63.0573) (35.5577, 63.0192) (35.6087, 62.9787) (35.6593, 62.9377) (35.7096, 62.8963) (35.7629, 62.8524) (35.8158, 62.808) (35.8682, 62.7632) (35.9237, 62.7158) (35.9787, 62.668) (36.0333, 62.6196) (36.1342, 62.5302) (36.2338, 62.4392) (36.332, 62.3467) knots 0 0 0 0 0.057795 0.057795 0.057795 0.089038 0.089038 0.089038 0.118617 0.118617 0.118617 0.14653 0.14653 0.14653 0.172778 0.172778 0.172778 0.19736 0.19736 0.19736 0.220277 0.220277 0.220277 0.241529 0.241529 0.241529 0.261115 0.261115 0.261115 0.279036 0.279036 0.279036 0.295292 0.295292 0.295292 0.309882 0.309882 0.309882 0.329164 0.329164 0.329164 0.333477 0.333477 0.333477 0.337694 0.337694 0.337694 0.34182 0.34182 0.34182 0.345864 0.345864 0.345864 0.349834 0.349834 0.349834 0.353742 0.353742 0.353742 0.3576 0.3576 0.3576 0.361424 0.361424 0.361424 0.365232 0.365232 0.365232 0.369048 0.369048 0.369048 0.372899 0.372899 0.372899 0.376819 0.376819 0.376819 0.380853 0.380853 0.380853 0.385052 0.385052 0.385052 0.389482 0.389482 0.389482 0.394225 0.394225 0.394225 0.399381 0.399381 0.399381 0.405067 0.405067 0.405067 0.411413 0.411413 0.411413 0.418548 0.418548 0.418548 0.426565 0.426565 0.426565 0.435472 0.435472 0.435472 0.445133 0.445133 0.445133 0.45436 0.45436 0.45436 0.5 0.5 0.5 0.54564 0.54564 0.54564 0.554867 0.554867 0.554867 0.564528 0.564528 0.564528 0.573435 0.573435 0.573435 0.581452 0.581452 0.581452 0.588587 0.588587 0.588587 0.594933 0.594933 0.594933 0.600619 0.600619 0.600619 0.605775 0.605775 0.605775 0.610518 0.610518 0.610518 0.614948 0.614948 0.614948 0.619147 0.619147 0.619147 0.623181 0.623181 0.623181 0.627101 0.627101 0.627101 0.630952 0.630952 0.630952 0.634768 0.634768 0.634768 0.638576 0.638576 0.638576 0.6424 0.6424 0.6424 0.646258 0.646258 0.646258 0.650166 0.650166 0.650166 0.654136 0.654136 0.654136 0.65818 0.65818 0.65818 0.662306 0.662306 0.662306 0.666523 0.666523 0.666523 0.670836 0.670836 0.670836 0.690118 0.690118 0.690118 0.704708 0.704708 0.704708 0.720964 0.720964 0.720964 0.738885 0.738885 0.738885 0.758471 0.758471 0.758471 0.779723 0.779723 0.779723 0.80264 0.80264 0.80264 0.827222 0.827222 0.827222 0.85347 0.85347 0.85347 0.881383 0.881383 0.881383 0.910962 0.910962 0.910962 0.942205 0.942205 0.942205 1 1 1 1
  arc A253 (37.3773, 65.1184) -> (37.7292, 66.2236) centre (0.0435, 77.6158) ccw
  spline S52 degree 3 poles (38.4791, 69.0893) (38.3455, 69.0707) (38.2117, 69.054) (38.0776, 69.0394) (38.0051, 69.0316) (37.9326, 69.0243) (37.86, 69.0177) (37.7912, 69.0115) (37.7224, 69.0059) (37.6536, 69.0009) (37.5886, 68.9961) (37.5236, 68.992) (37.4586, 68.9884) (37.3974, 68.9851) (37.3362, 68.9822) (37.275, 68.98) (37.2177, 68.9778) (37.1604, 68.9762) (37.103, 68.9751) (37.0495, 68.9741) (36.9961, 68.9735) (36.9426, 68.9734) (36.893, 68.9734) (36.8434, 68.9737) (36.7938, 68.9745) (36.7481, 68.9753) (36.7024, 68.9764) (36.6568, 68.978) (36.615, 68.9794) (36.5732, 68.9812) (36.5314, 68.9833) (36.4935, 68.9853) (36.4557, 68.9876) (36.4178, 68.9902) (36.3839, 68.9926) (36.3499, 68.9952) (36.316, 68.9982) (36.2712, 69.0022) (36.2264, 69.0068) (36.1817, 69.0118) (36.1717, 69.0129) (36.1617, 69.014) (36.1517, 69.015) (36.1419, 69.016) (36.1321, 69.0169) (36.1223, 69.0177) (36.1127, 69.0185) (36.1031, 69.0192) (36.0935, 69.0199) (36.0841, 69.0205) (36.0746, 69.021) (36.0652, 69.0215) (36.056, 69.0219) (36.0467, 69.0222) (36.0374, 69.0225) (36.0283, 69.0227) (36.0192, 69.0229) (36.0101, 69.0229) (36.0011, 69.0229) (35.9921, 69.0229) (35.9831, 69.0227) (35.9742, 69.0225) (35.9652, 69.0223) (35.9563, 69.0219) (35.9474, 69.0215) (35.9386, 69.021) (35.9297, 69.0203) (35.9208, 69.0197) (35.912, 69.0189) (35.9031, 69.018) (35.8942, 69.0171) (35.8852, 69.0161) (35.8763, 69.0149) (35.8673, 69.0136) (35.8582, 69.0122) (35.8492, 69.0107) (35.8399, 69.009) (35.8307, 69.0073) (35.8215, 69.0053) (35.8119, 69.0032) (35.8024, 69.0009) (35.7929, 68.9984) (35.7829, 68.9957) (35.773, 68.9928) (35.7632, 68.9896) (35.7526, 68.9862) (35.7422, 68.9825) (35.7319, 68.9785) (35.7207, 68.9741) (35.7096, 68.9693) (35.6988, 68.9641) (35.6868, 68.9584) (35.675, 68.9523) (35.6635, 68.9456) (35.6507, 68.9382) (35.6382, 68.9301) (35.6262, 68.9215) (35.6126, 68.9118) (35.5996, 68.9014) (35.5872, 68.8902) (35.5733, 68.8777) (35.5602, 68.8643) (35.548, 68.8501) (35.5345, 68.8343) (35.5221, 68.8176) (35.511, 68.8) (35.4989, 68.7809) (35.4883, 68.7609) (35.4796, 68.7401) (35.4713, 68.7202) (35.4647, 68.6996) (35.4585, 68.679) (35.4279, 68.5769) (35.4059, 68.4725) (35.379, 68.3695) (35.352, 68.2665) (35.32, 68.1649) (35.2968, 68.0608) (35.292, 68.0398) (35.2877, 68.0186) (35.2852, 67.9973) (35.2826, 67.9749) (35.282, 67.9522) (35.2832, 67.9296) (35.2843, 67.9089) (35.2869, 67.8882) (35.291, 67.8678) (35.2946, 67.8494) (35.2995, 67.8313) (35.3055, 67.8136) (35.3109, 67.7978) (35.3171, 67.7823) (35.3242, 67.7672) (35.3304, 67.7538) (35.3374, 67.7407) (35.3449, 67.728) (35.3517, 67.7165) (35.3589, 67.7054) (35.3665, 67.6945) (35.3735, 67.6847) (35.3808, 67.6751) (35.3884, 67.6658) (35.3954, 67.6573) (35.4027, 67.6489) (35.4102, 67.6408) (35.4172, 67.6332) (35.4244, 67.6258) (35.4319, 67.6186) (35.4389, 67.6117) (35.4461, 67.6051) (35.4534, 67.5986) (35.4604, 67.5923) (35.4676, 67.5862) (35.4749, 67.5803) (35.482, 67.5745) (35.4892, 67.5689) (35.4965, 67.5633) (35.5037, 67.5579) (35.5109, 67.5526) (35.5183, 67.5475) (35.5256, 67.5423) (35.5329, 67.5373) (35.5404, 67.5324) (35.5478, 67.5275) (35.5553, 67.5227) (35.5628, 67.518) (35.5704, 67.5133) (35.578, 67.5087) (35.5857, 67.5042) (35.5935, 67.4996) (35.6013, 67.4952) (35.6092, 67.4908) (35.6172, 67.4864) (35.6252, 67.482) (35.6332, 67.4778) (35.6414, 67.4735) (35.6497, 67.4692) (35.658, 67.4651) (35.6664, 67.4608) (35.6749, 67.4567) (35.6834, 67.4526) (35.6921, 67.4485) (35.7008, 67.4444) (35.7095, 67.4404) (35.7185, 67.4363) (35.7275, 67.4323) (35.7365, 67.4283) (35.7457, 67.4243) (35.755, 67.4204) (35.7643, 67.4165) (35.8057, 67.3989) (35.847, 67.381) (35.888, 67.3625) (35.919, 67.3485) (35.9499, 67.3342) (35.9807, 67.3196) (36.0149, 67.3034) (36.0491, 67.2868) (36.0831, 67.27) (36.1205, 67.2514) (36.1578, 67.2325) (36.195, 67.2133) (36.2356, 67.1922) (36.276, 67.1709) (36.3162, 67.1491) (36.3598, 67.1255) (36.4032, 67.1016) (36.4464, 67.0772) (36.493, 67.0509) (36.5393, 67.0242) (36.5854, 66.9972) (36.6349, 66.9681) (36.6841, 66.9386) (36.733, 66.9087) (36.7853, 66.8767) (36.8373, 66.8443) (36.8889, 66.8114) (36.9439, 66.7764) (36.9985, 66.741) (37.0528, 66.705) (37.1104, 66.6669) (37.1676, 66.6283) (37.2245, 66.5892) (37.2846, 66.5479) (37.3443, 66.5061) (37.4036, 66.4637) (37.5134, 66.3854) (37.6219, 66.3052) (37.7292, 66.2236) knots 0 0 0 0 0.057795 0.057795 0.057795 0.089038 0.089038 0.089038 0.118617 0.118617 0.118617 0.14653 0.14653 0.14653 0.172778 0.172778 0.172778 0.19736 0.19736 0.19736 0.220277 0.220277 0.220277 0.241529 0.241529 0.241529 0.261115 0.261115 0.261115 0.279036 0.279036 0.279036 0.295292 0.295292 0.295292 0.309882 0.309882 0.309882 0.329164 0.329164 0.329164 0.333477 0.333477 0.333477 0.337694 0.337694 0.337694 0.34182 0.34182 0.34182 0.345864 0.345864 0.345864 0.349834 0.349834 0.349834 0.353742 0.353742 0.353742 0.3576 0.3576 0.3576 0.361424 0.361424 0.361424 0.365232 0.365232 0.365232 0.369048 0.369048 0.369048 0.372899 0.372899 0.372899 0.376819 0.376819 0.376819 0.380853 0.380853 0.380853 0.385052 0.385052 0.385052 0.389482 0.389482 0.389482 0.394225 0.394225 0.394225 0.399381 0.399381 0.399381 0.405067 0.405067 0.405067 0.411413 0.411413 0.411413 0.418548 0.418548 0.418548 0.426565 0.426565 0.426565 0.435472 0.435472 0.435472 0.445133 0.445133 0.445133 0.45436 0.45436 0.45436 0.5 0.5 0.5 0.54564 0.54564 0.54564 0.554867 0.554867 0.554867 0.564528 0.564528 0.564528 0.573435 0.573435 0.573435 0.581452 0.581452 0.581452 0.588587 0.588587 0.588587 0.594933 0.594933 0.594933 0.600619 0.600619 0.600619 0.605775 0.605775 0.605775 0.610518 0.610518 0.610518 0.614948 0.614948 0.614948 0.619147 0.619147 0.619147 0.623181 0.623181 0.623181 0.627101 0.627101 0.627101 0.630952 0.630952 0.630952 0.634768 0.634768 0.634768 0.638576 0.638576 0.638576 0.6424 0.6424 0.6424 0.646258 0.646258 0.646258 0.650166 0.650166 0.650166 0.654136 0.654136 0.654136 0.65818 0.65818 0.65818 0.662306 0.662306 0.662306 0.666523 0.666523 0.666523 0.670836 0.670836 0.670836 0.690118 0.690118 0.690118 0.704708 0.704708 0.704708 0.720964 0.720964 0.720964 0.738885 0.738885 0.738885 0.758471 0.758471 0.758471 0.779723 0.779723 0.779723 0.80264 0.80264 0.80264 0.827222 0.827222 0.827222 0.85347 0.85347 0.85347 0.881383 0.881383 0.881383 0.910962 0.910962 0.910962 0.942205 0.942205 0.942205 1 1 1 1
  arc A254 (38.4791, 69.0893) -> (38.7136, 70.2252) centre (0.0435, 77.6158) ccw